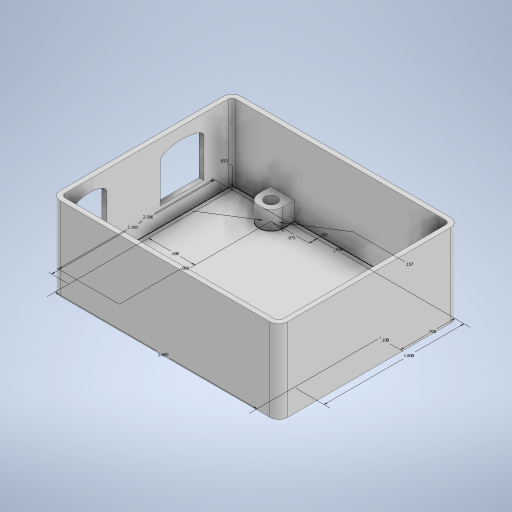
# Autodesk Inventor part: ArduinoHolder-v3
Saved by Autodesk Inventor 2023 (Build 270158030, 158C)
## iProperties
Created: 2024-03-14
Part Number: ArduinoHolder-v3
Material: Generic
Document SubType Name: Modeling
Designer: lvrectanus0
Density: 1 g/cm^3
Appearance: Default
Author: lvrectanus0
Autodesk Inventor part; units mm, degrees
ref_plane "YZ Plane" through (0, 0, 0) normal (1, 0, 0) x (0, 1, 0)
ref_plane "XZ Plane" through (0, 0, 0) normal (0, 1, 0) x (-1, 0, 0)
ref_plane "XY Plane" through (0, 0, 0) normal (0, 0, 1) x (1, 0, 0)
sketch "Sketch1" plane through (0, 0, 0) normal (0, 1, 0) x (-1, 0, 0)
  circle A0 centre (-15.24, 2.54) radius 2
  circle A1 centre (-66.04, 17.78) radius 2
  circle A2 centre (-66.04, 45.72) radius 2
  line L0 (0, 0) -> (-68.58, 0) construction
  line L1 (-68.58, 0) -> (-68.58, 53.34) construction
  line L2 (-68.58, 53.34) -> (0, 53.34) construction
  line L3 (0, 53.34) -> (0, 0) construction
  line L4 (-68.58, -1.27) -> (0, -1.27)
  line L5 (1.27, 0) -> (1.27, 53.34)
  line L6 (0, 54.61) -> (-68.58, 54.61)
  line L7 (-69.85, 53.34) -> (-69.85, 0)
  arc A3 (0, -1.27) -> (1.27, 0) centre (0, 0) ccw
  arc A4 (-69.85, 0) -> (-68.58, -1.27) centre (-68.58, 0) ccw
  arc A5 (-68.58, 54.61) -> (-69.85, 53.34) centre (-68.58, 53.34) ccw
  arc A6 (1.27, 53.34) -> (0, 54.61) centre (0, 53.34) ccw
  arc A7 (-11.335, 2.54) -> (-19.145, 2.54) centre (-15.24, 2.54) ccw
  arc A8 (-66.04, 41.815) -> (-66.04, 49.625) centre (-66.04, 45.72) ccw
  arc A9 (-66.04, 13.875) -> (-66.04, 21.685) centre (-66.04, 17.78) ccw
  line L8 (-11.335, 2.54) -> (-19.145, 2.54) construction
  line L9 (-19.145, 2.54) -> (-19.145, -1.27)
  line L10 (-19.145, -1.27) -> (-11.335, -1.27)
  line L11 (-11.335, -1.27) -> (-11.335, 2.54)
  line L12 (-66.04, 13.875) -> (-69.85, 13.875)
  line L13 (-69.85, 13.875) -> (-69.85, 21.685)
  line L14 (-69.85, 21.685) -> (-66.04, 21.685)
  line L15 (-66.04, 21.685) -> (-66.04, 13.875) construction
  line L16 (-66.04, 41.815) -> (-69.85, 41.815)
  line L17 (-69.85, 41.815) -> (-69.85, 49.625)
  line L18 (-69.85, 49.625) -> (-66.04, 49.625)
  line L19 (-66.04, 49.625) -> (-66.04, 41.815) construction
  line L20 (-11.335, 54.61) -> (-19.145, 54.61)
  circle A10 centre (-13.97, 50.8) radius 2
  circle A11 centre (-13.97, 50.8) radius 3.905 construction
  arc A12 (-17.875, 50.8) -> (-10.065, 50.8) centre (-13.97, 50.8) ccw
  line L21 (-17.875, 50.8) -> (-17.875, 54.61)
  line L22 (-10.065, 50.8) -> (-10.065, 54.61)
  point P0 (-15.24, 2.54)
  dimension "d0" = 4
  dimension "d4" = 15.24
  dimension "d5" = 2.54
  dimension "d6" = 17.78
  dimension "d7" = 66.04
  dimension "d8" = 45.72
  dimension "d10" = 2.54
  dimension "d12" = 1.27
  dimension "d13" = 1.27
  dimension "d14" = 1.905
  dimension "d51" = 53.34
  dimension "d52" = 50.8
  dimension "d54" = 1.27
  constraints: 46 end point, 18 point on circle, 14 tangent, 13 centre point, 11 parallel, 10 equal radius, 8 point on line, 7 perpendicular, 4 horizontal, 2 coincident, 1 horizontal alignment, 1 midpoint, 1 vertical alignment, 3 other
  measures "d0" diameter of A0
  measures "d4" horizontal distance of A0.centre L0.start
  measures "d5" vertical distance of A0.centre L0.start
  measures "d6" vertical distance of A1.centre L0.start
  measures "d7" horizontal distance of L0.start A1.centre
  measures "d8" vertical distance of L0.start A2.centre
  measures "d10" distance from line of L1 A1.centre
  measures "d12" distance between parallel lines of L0 L4
  measures "d13" radius of A3
  measures "d14" radial gap between concentric circles of A0 A7
  measures "d51" distance of A6.centre L0.start
  measures "d52" vertical distance of A10.centre L0.start
  measures "d54" horizontal distance of A10.centre A0.centre
extrude "Extrusion1" add sketch "Sketch1" along normal blind 6 contours L9 A7 L11 L4 | L7 L14 A9 L12 | L7 L18 A8 L16 | L22 A12 L21 L6
extrude "Extrusion2" add sketch "Sketch1" against normal blind 2
sketch "Sketch2" plane through (0, -2, 0) normal (0, -1, 0) x (1, 0, 0)
  line L0 (68.58, 54.61) -> (0, 54.61) projected
  arc A0 (0, 54.61) -> (-1.27, 53.34) centre (0, 53.34) ccw projected
  line L1 (-1.27, 53.34) -> (-1.27, 0) projected
  arc A1 (-1.27, 0) -> (0, -1.27) centre (0, 0) ccw projected
  line L2 (0, -1.27) -> (68.58, -1.27) projected
  arc A2 (68.58, -1.27) -> (69.85, 0) centre (68.58, 0) ccw projected
  line L3 (69.85, 0) -> (69.85, 53.34) projected
  arc A3 (69.85, 53.34) -> (68.58, 54.61) centre (68.58, 53.34) ccw projected
  line L4 (68.58, -2.8575) -> (0, -2.8575)
  arc A4 (-2.8575, 0) -> (0, -2.8575) centre (0, 0) ccw
  line L5 (-2.8575, 0) -> (-2.8575, 53.34)
  arc A5 (0, 56.1975) -> (-2.8575, 53.34) centre (0, 53.34) ccw
  line L6 (0, 56.1975) -> (68.58, 56.1975)
  arc A6 (71.4375, 53.34) -> (68.58, 56.1975) centre (68.58, 53.34) ccw
  line L7 (71.4375, 53.34) -> (71.4375, 0)
  arc A7 (68.58, -2.8575) -> (71.4375, 0) centre (68.58, 0) ccw
  point P0 (0, 0)
  dimension "d19" = 1.5875
  constraints: 8 end point, 8 point on circle, 4 centre point, 7 other
  measures "d19" distance between parallel lines of L2 L4
extrude "Extrusion3" add sketch "Sketch2" against normal blind 27.05
sketch "Sketch4" plane through (-2.8575, -2, 0) normal (-1, 0, 0) x (0, 0, 1)
  line L0 (0, 2) -> (53.34, 2) projected
  line L1 (0, 27.05) -> (53.34, 27.05) projected
  line L2 (50.8, 20.7) -> (39.6875, 20.7) construction
  line L3 (39.6875, 20.7) -> (39.6875, 8)
  ellipse E0 centre (45.2438, 20.7) end of major axis (50.8, 20.7) minor radius 2.54 (50.8, 20.7) -> (39.6875, 20.7) ccw
  ellipse E1 centre (45.2438, 20.7) end of major axis (50.8, 20.7) minor radius 2.54 (39.6875, 20.7) -> (50.8, 20.7) ccw construction
  line L4 (7.9375, 8) -> (7.9375, 20.7)
  line L5 (22.225, 8) -> (22.225, 20.7)
  ellipse E2 centre (15.0813, 20.7) end of major axis (22.225, 20.7) minor radius 2.54 (22.225, 20.7) -> (7.9375, 20.7) ccw
  line L6 (7.9375, 8) -> (22.225, 8)
  line L7 (50.8, 20.7) -> (50.8, 8)
  line L8 (50.8, 8) -> (39.6875, 8)
  line L9 (50.8, 8) -> (54.61, 8) projected
  line L10 (54.61, 8) -> (50.8, 8) projected
  line L11 (50.8, 8) -> (50.8, 8) projected
  line L12 (48.8, 8) -> (52.8, 8) projected
  line L13 (2.54, 8) -> (-1.27, 8) projected
  line L14 (-1.27, 8) -> (2.54, 8) projected
  line L15 (2.54, 8) -> (2.54, 8) projected
  line L16 (0.54, 8) -> (4.54, 8) projected
  line L17 (53.34, 0) -> (53.34, 27.05) projected
  point P0 (2.54, 2)
  point P1 (2.54, 2)
  point P2 (2.54, 2)
  point P3 (2.54, 2)
  dimension "d26" = 2.54
  dimension "d29" = 2.54
  dimension "d25" = 11.1125
  dimension "d27" = 7.9375
  dimension "d28" = 14.2875
  dimension "d56" = 2.54
  dimension "d57" = 12.7
  constraints: 14 end point, 5 horizontal alignment, 5 vertical, 3 horizontal, 3 parallel, 1 midpoint, 12 other
  measures "d25" distance of L2.start L2.end
  measures "d27" horizontal distance of L4.start L0.start
  measures "d28" distance of L4.start L5.start
  measures "d56" distance between parallel lines of L17 L7
  measures "d57" distance of L5.start L5.end
extrude "Extrusion5" cut sketch "Sketch4" against normal up to surface (1.5875 mm away)
sketch "Sketch6" plane through (0, 0, 0) normal (0, 1, 0) x (1, 0, 0)
  line L0 (28.6568, -13.7506) -> (43.0772, -34.6602)
  point P0 (0, 0)
  dimension "d50" = 25.4
  constraints: 2 end point
  measures "d50" distance of L0.start L0.end
sketch "Sketch7" plane through (-2.8575, -2, 0) normal (-1, 0, 0) x (0, 0, 1)
  line L0 (0, 0) -> (0, 27.05) projected
  line L1 (0, 0) -> (-8.89, 0)
  line L2 (-8.89, 0) -> (-21.1351, -14.5931)
  line L3 (-21.1351, -14.5931) -> (-21.1351, -17.1331)
  line L4 (-21.1351, -17.1331) -> (11.9427, -44.8887)
  line L5 (53.34, 0) -> (0, 0) construction
  line L6 (26.67, 0) -> (26.67, -45.2204) construction
  line L7 (-8.89, 0) -> (25.1607, -28.5719) construction
  point P0 (0, 2)
  dimension "d58" = 8.89
  dimension "d59" = 19.05
  dimension "d60" = 130
  dimension "d61" = 2.54
  dimension "d62" = 43.18
  dimension "d63" = 130
  constraints: 12 end point, 3 perpendicular, 1 horizontal, 1 midpoint, 1 vertical
  measures "d58" distance of L0.start L1.end
  measures "d59" distance of L1.end L2.end
  measures "d60" angle of L2 L1
  measures "d61" distance of L2.end L3.end
  measures "d62" distance of L3.end L4.end
  measures "d63" angle of L4 L3
body "Solid1"
